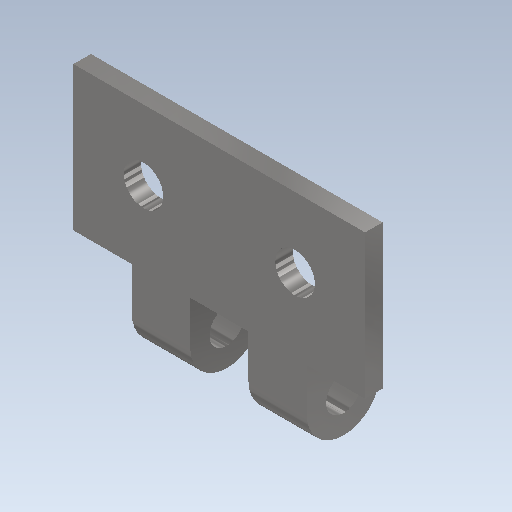
# Autodesk Inventor part: 1HHKS25
Saved by Autodesk Inventor 2021 (Build 250183000, 183)
## iProperties
Part Number: 1HHKS25
Material: ステンレス鋼
Catalog Web Link: www.cadenas.de
Description: HHKS-1-Hinges
Vendor: MISUMI
Document SubType Name: Modeling
Designer: partserver
Manufacturer: MISUMI
Mass: 5.64576 g
Surface Area: 11.189 cm^2
Volume: 0.70572 cm^3
Density: 8 g/cm^3
Appearance: 半つや出し
Category: PARTsolutions
Company: MISUMI
PSOL_IDENT_0: {$CADENAS_DATA\23d-libs\misumi\metric\43_levers_knobs\parts_hhks\hhks_1.prj},147 {VTYP=3D},{NB=1HHKS
PSOL_IDENT_1: 25},{LINA=1HHKS25},{NN=HHKS-1},{DATE=30.03.2018 07:16:18},{GEOMDATE=17.02.2014},{VERSION=},{LINEID=1
PSOL_IDENT_2: 0},{WBVAR=L},{WBNUMERIC=L}  {NB=1HHKS25},{LINA=1HHKS25},{KT=DUMMY},{PN=HHKS25},{MAT=304 Stainless St
PSOL_IDENT_3: eel},{L=25},{LL=6.0},{L1=13},{L2=0},{L3=0},{NOD=3},{AL=29.4},{WEIGHT=13}
NB: 1HHKS25
NN: HHKS-1
NT: Hinges
NBSYN: 1$PN.
LINA: 1HHKS25
CATALOG: Misumi
MAT: 304 Stainless Steel
L: 25
SUPPLIER: MISUMI
ARTICLENO: 1HHKS25
BOMINFO: 1HHKS25
CREATOR: CADENAS GmbH
Title: 1HHKS25
Author: Cadenas PARTsolutions
Comments: Hinges
Autodesk Inventor part; units mm, degrees
sketch "Sketch_10" plane through (0, 0, 0) normal (0, 1, 0) x (-1, 0, 0)
  line L0 (0, -3.65) -> (-5, -3.65)
  line L1 (-5, -3.65) -> (-5, -3.15)
  line L2 (-5, -3.15) -> (-10, -3.15)
  line L3 (-10, -3.15) -> (-10, -3.65)
  line L4 (-10, -3.65) -> (-15, -3.65)
  line L5 (-15, -3.65) -> (-15, -3.15)
  line L6 (-15, -3.15) -> (-20, -3.15)
  line L7 (-20, -3.15) -> (-20, -3.65)
  line L8 (-20, -3.65) -> (-25, -3.65)
  line L9 (-25, -3.65) -> (-25, -16)
  line L10 (-25, -16) -> (0, -16)
  line L11 (0, -16) -> (0, -3.65)
  constraints: 24 end point
extrude "Extrusion1" add sketch "Sketch_10" along normal blind 1.5
sketch "Sketch_2" plane through (5, 0, 0) normal (1, 0, 0) x (0, 0, -1)
  arc A0 (3.15, 3.15) -> (0, 0) centre (0, 3.15) ccw
  line L0 (0, 0) -> (10.6667, 0)
  line L1 (10.6667, 0) -> (10.6667, 1.5)
  line L2 (10.6667, 1.5) -> (3.15, 1.5)
  line L3 (3.15, 1.5) -> (3.15, 3.15)
  circle A1 centre (0, 3.15) radius 1.5
  constraints: 8 end point, 2 centre point, 2 point on circle
extrude "Extrusion2" add sketch "Sketch_2" along normal blind 5
sketch "Sketch_3" plane through (15, 0, 0) normal (1, 0, 0) x (0, 0, -1)
  arc A0 (3.15, 3.15) -> (0, 0) centre (0, 3.15) ccw
  line L0 (0, 0) -> (10.6667, 0)
  line L1 (10.6667, 0) -> (10.6667, 1.5)
  line L2 (10.6667, 1.5) -> (3.15, 1.5)
  line L3 (3.15, 1.5) -> (3.15, 3.15)
  circle A1 centre (0, 3.15) radius 1.5
  constraints: 8 end point, 2 centre point, 2 point on circle
extrude "Extrusion3" add sketch "Sketch_3" along normal blind 5
sketch "Sketch4" plane through (0, 0, 0) normal (0, -1, 0) x (1, 0, 0)
  point P0 (6, -10)
hole "Hole1" at (6, 0, -10) direction (0, 1, 0) diameter 3.4 depth 2
sketch "Sketch5" plane through (0, 0, 0) normal (0, -1, 0) x (1, 0, 0)
  point P0 (19, -10)
hole "Hole2" at (19, 0, -10) direction (0, 1, 0) diameter 3.4 depth 2
ref_plane "1_XY" through (0, 3.15, 0) normal (1, 0, 0) x (0, 0, -1)
ref_plane "1_YZ" through (0, 3.15, 0) normal (0, 0, -1) x (0, 1, 0)
ref_plane "1_ZX" through (0, 3.15, 0) normal (0, 1, 0) x (1, 0, 0)
ref_plane "11_XY" through (0, 3.15, 0) normal (1, 0, 0) x (0, 0, -1)
ref_plane "11_YZ" through (0, 3.15, 0) normal (0, 0, -1) x (0, 1, 0)
ref_plane "11_ZX" through (0, 3.15, 0) normal (0, 1, 0) x (1, 0, 0)
body "Solid1"
